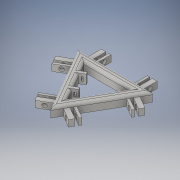
# Autodesk Inventor part: Test End effector
Saved by Autodesk Inventor 2016 (Build 200138000, 138)
## iProperties
Created: 2018-08-18
Part Number: Test End effector
Material: Generic
Document SubType Name: Modeling
Designer: Jorian Bruslind
Density: 1 g/cm^3
Appearance: Default
Author: Jorian Bruslind
Autodesk Inventor part; units mm, degrees
ref_plane "YZ Plane" through (0, 0, 0) normal (1, 0, 0) x (0, 1, 0)
ref_plane "XZ Plane" through (0, 0, 0) normal (0, 1, 0) x (-1, 0, 0)
ref_plane "XY Plane" through (0, 0, 0) normal (0, 0, 1) x (1, 0, 0)
sketch "Sketch1" plane through (0, 0, 0) normal (0, 1, 0) x (-1, 0, 0)
  line L0 (0, 46.188) -> (40, -23.094)
  line L1 (40, -23.094) -> (-40, -23.094)
  line L2 (-40, -23.094) -> (0, 46.188)
  line L3 (0, 28.8675) -> (25, -14.4338)
  line L4 (25, -14.4338) -> (-25, -14.4338)
  line L5 (-25, -14.4338) -> (0, 28.8675)
  point P0 (0, 0)
  point P1 (0, 0)
  point P2 (0, 0)
  dimension "d18" = 80
  dimension "d19" = 50
  constraints: 12 end point, 2 coincident, 14 other
  measures "d18" distance of L0.end L1.end
  measures "d19" distance of L3.end L4.end
extrude "Extrusion1" add sketch "Sketch1" along normal blind 10
sketch "Sketch5" plane through (40, 0, -23.094) normal (0.8660254, 0, 0.5) x (0.5, 0, -0.8660254)
  line L0 (0, 0) -> (-80, 0) projected
  line L1 (0, 0) -> (-10, 0)
  line L2 (-10, 0) -> (-15, 0)
  line L3 (-15, 0) -> (-15, 7)
  line L4 (-15, 7) -> (-10, 7)
  line L5 (-10, 7) -> (-10, 0)
  line L6 (-15, 0) -> (-18, 0)
  line L7 (-18, 0) -> (-20.5, 0)
  line L8 (-20.5, 0) -> (-20.5, 7)
  line L9 (-20.5, 7) -> (-18, 7)
  line L10 (-18, 7) -> (-18, 0)
  line L11 (-80, 0) -> (-70, 0)
  line L12 (-80, 0) -> (-40, 0) projected
  line L13 (-70, 0) -> (-65, 0)
  line L14 (-65, 0) -> (-65, 7)
  line L15 (-65, 7) -> (-70, 7)
  line L16 (-70, 7) -> (-70, 0)
  line L17 (-65, 0) -> (-62, 0)
  line L18 (-62, 0) -> (-59.5, 0)
  line L19 (-59.5, 0) -> (-59.5, 7)
  line L20 (-59.5, 7) -> (-62, 7)
  line L21 (-62, 7) -> (-62, 0)
  dimension "d44" = 10
  dimension "d45" = 5
  dimension "d46" = 7
  dimension "d47" = 3
  dimension "d48" = 2.5
  dimension "d49" = 10
  dimension "d50" = 5
  dimension "d51" = 7
  dimension "d52" = 3
  dimension "d53" = 2.5
  dimension "d54" = 7
  constraints: 40 end point, 8 parallel, 4 horizontal, 4 perpendicular, 4 point on line
  measures "d44" distance of L0.start L1.end
  measures "d45" distance of L3.end L4.end
  measures "d46" distance of L2.end L3.end
  measures "d47" distance of L2.end L6.end
  measures "d48" distance of L8.end L9.end
  measures "d49" distance of L0.end L11.end
  measures "d50" distance of L15.end L14.end
  measures "d51" distance of L14.end L13.end
  measures "d52" distance of L13.end L17.end
  measures "d53" distance of L20.end L19.end
  measures "d54" distance of L19.end L18.end
extrude "Extrusion3" add sketch "Sketch5" along normal blind 15
sketch "Sketch6" plane through (5, 0, 37.5278) normal (-0.5, 0, 0.8660254) x (0.8660254, 0, 0.5)
  line L0 (15, 0) -> (15, 7) projected
  line L1 (15, 3.5) -> (7.5, 3.5)
  circle A0 centre (7.5, 3.5) radius 2.25
  point P0 (-23.094, 0)
  dimension "d57" = 7.5
  dimension "d58" = 4.5
  constraints: 2 end point, 1 centre point, 1 coincident, 1 horizontal, 1 midpoint
  measures "d57" distance of L1.start L1.end
  measures "d58" diameter of A0
extrude "Extrusion4" cut sketch "Sketch6" against normal blind 60
sketch "Sketch7" plane through (0, 0, 46.188) normal (-0.8660254, 0, 0.5) x (0.5, 0, 0.8660254)
  line L0 (-80, 0) -> (-40, 0) projected
  line L1 (-80, 0) -> (-70, 0)
  line L2 (0, 0) -> (0, 10) projected
  line L3 (0, 0) -> (-10, 0)
  line L4 (0, 0) -> (-80, 0) projected
  line L5 (-70, 0) -> (-65, 0)
  line L6 (-65, 0) -> (-65, 7)
  line L7 (-65, 7) -> (-70, 7)
  line L8 (-70, 7) -> (-70, 0)
  line L9 (-65, 0) -> (-62, 0)
  line L10 (-65, 0) -> (-15, 0) projected
  line L11 (-62, 0) -> (-59.5, 0)
  line L12 (-59.5, 0) -> (-59.5, 7)
  line L13 (-59.5, 7) -> (-62, 7)
  line L14 (-62, 7) -> (-62, 0)
  line L15 (-10, 0) -> (-15, 0)
  line L16 (-15, 0) -> (-15, 7)
  line L17 (-15, 7) -> (-10, 7)
  line L18 (-10, 7) -> (-10, 0)
  line L19 (-15, 0) -> (-18, 0)
  line L20 (-32.5, 7) -> (-19.5096, 7) projected
  line L21 (-18, 0) -> (-20.5, 0)
  line L22 (-20.5, 0) -> (-20.5, 7)
  line L23 (-20.5, 7) -> (-18, 7)
  line L24 (-18, 7) -> (-18, 0)
  dimension "d61" = 10
  dimension "d62" = 10
  dimension "d63" = 5
  dimension "d64" = 7
  dimension "d65" = 3
  dimension "d66" = 2.5
  dimension "d67" = 7
  dimension "d68" = 5
  dimension "d69" = 7
  dimension "d70" = 3
  dimension "d71" = 2.5
  constraints: 40 end point, 8 parallel, 5 point on line, 4 horizontal, 4 perpendicular
  measures "d61" distance of L0.start L1.end
  measures "d62" distance of L2.start L3.end
  measures "d63" distance of L7.end L6.end
  measures "d64" distance of L6.end L5.end
  measures "d65" distance of L5.end L9.end
  measures "d66" distance of L13.end L12.end
  measures "d67" distance of L12.end L11.end
  measures "d68" distance of L16.end L17.end
  measures "d69" distance of L15.end L16.end
  measures "d70" distance of L15.end L19.end
  measures "d71" distance of L22.end L23.end
extrude "Extrusion5" add sketch "Sketch7" along normal blind 15
sketch "Sketch8" plane through (-35, 0, -14.4338) normal (-0.5, 0, -0.8660254) x (-0.8660254, 0, 0.5)
  line L0 (15, 7) -> (15, 0) projected
  line L1 (15, 3.5) -> (7.5, 3.5)
  circle A0 centre (7.5, 3.5) radius 2.25
  point P0 (-23.094, 0)
  dimension "d74" = 7.5
  dimension "d75" = 90
  dimension "d76" = 4.5
  constraints: 2 end point, 1 centre point, 1 coincident, 1 midpoint
  measures "d74" distance of L1.start L1.end
  measures "d75" angle of L0 L1
  measures "d76" diameter of A0
extrude "Extrusion6" cut sketch "Sketch8" against normal blind 60
sketch "Sketch9" plane through (40, 0, -23.094) normal (0, 0, -1) x (-1, 0, 0)
  line L0 (0, 0) -> (0, 10) projected
  line L1 (0, 0) -> (10, 0)
  line L2 (10.25, 0) -> (-2.7404, 0) projected
  line L3 (80, 0) -> (80, 10) projected
  line L4 (80, 0) -> (70, 0)
  line L5 (71, 0) -> (83.9904, 0) projected
  line L6 (10.25, 0) -> (15.25, 0)
  line L7 (15.25, 0) -> (15.25, 7)
  line L8 (15.25, 7) -> (10.25, 7)
  line L9 (10.25, 7) -> (10.25, 0)
  line L10 (15.25, 0) -> (18.25, 0)
  line L11 (18.0096, 0) -> (16.7596, 0) projected
  line L12 (32.5, 7) -> (19.5096, 7) projected
  line L13 (18.0096, 0) -> (20.5096, 0)
  line L14 (20.5096, 0) -> (20.5096, 7)
  line L15 (20.5096, 7) -> (18.0096, 7)
  line L16 (18.0096, 7) -> (18.0096, 0)
  line L17 (70, 0) -> (65, 0)
  line L18 (65, 0) -> (65, 7)
  line L19 (65, 7) -> (70, 7)
  line L20 (70, 7) -> (70, 0)
  line L21 (65, 0) -> (62, 0)
  line L22 (62, 0) -> (59.5, 0)
  line L23 (59.5, 0) -> (59.5, 7)
  line L24 (59.5, 7) -> (62, 7)
  line L25 (62, 7) -> (62, 0)
  point P0 (40, 0)
  dimension "d79" = 10
  dimension "d80" = 10
  dimension "d81" = 5
  dimension "d82" = 7
  dimension "d83" = 3
  dimension "d84" = 2.5
  dimension "d85" = 5
  dimension "d86" = 7
  dimension "d87" = 3
  dimension "d88" = 2.5
  dimension "d89" = 7
  constraints: 40 end point, 8 parallel, 5 horizontal, 4 perpendicular, 3 collinear, 1 point on line
  measures "d79" distance of L0.start L1.end
  measures "d80" distance of L3.start L4.end
  measures "d81" distance of L8.end L7.end
  measures "d82" distance of L7.end L6.end
  measures "d83" distance of L6.end L10.end
  measures "d84" distance of L15.end L14.end
  measures "d85" distance of L18.end L19.end
  measures "d86" distance of L17.end L18.end
  measures "d87" distance of L17.end L21.end
  measures "d88" distance of L23.end L24.end
  measures "d89" distance of L22.end L23.end
extrude "Extrusion7" add sketch "Sketch9" along normal blind 15
sketch "Sketch10" plane through (29.75, 0, -23.094) normal (1, 0, 0) x (0, 0, -1)
  line L0 (15, 7) -> (15, 0) projected
  line L1 (15, 3.5) -> (7.5, 3.5)
  circle A0 centre (7.5, 3.5) radius 2.25
  point P0 (-23.094, 0)
  dimension "d92" = 7.5
  dimension "d93" = 4.5
  constraints: 2 end point, 1 centre point, 1 coincident, 1 horizontal, 1 midpoint
  measures "d92" distance of L1.start L1.end
  measures "d93" diameter of A0
extrude "Extrusion8" cut sketch "Sketch10" against normal blind 60
sketch "Sketch11" plane through (-25, 0, -14.4338) normal (0.8660254, 0, -0.5) x (-0.5, 0, -0.8660254)
  line L0 (-25, 0) -> (-16, 0)
  line L1 (0, 0) -> (-50, 0) projected
  line L2 (-25, 0) -> (-16, 0) construction
  line L3 (-25, 0) -> (-34, 0)
  line L4 (-25, 0) -> (-16, 0) construction
  line L5 (-50, 10) -> (0, 10) projected
  line L6 (-16, 0) -> (-13, 0)
  line L7 (-13, 0) -> (-13, 10)
  line L8 (-13, 10) -> (-16, 10)
  line L9 (-16, 10) -> (-16, 0)
  line L10 (-34, 0) -> (-37, 0)
  line L11 (-37, 0) -> (-37, 10)
  line L12 (-37, 10) -> (-34, 10)
  line L13 (-34, 10) -> (-34, 0)
  dimension "d97" = 9
  dimension "d98" = 0
  dimension "d99" = 9
  dimension "d100" = 180
  dimension "d101" = 3
  dimension "d102" = 3
  constraints: 24 end point, 4 collinear, 4 horizontal, 4 parallel, 2 perpendicular, 2 point on line
  measures "d97" distance of L0.start L0.end
  measures "d98" distance between parallel lines of L2 L0
  measures "d99" distance of L0.start L3.end
  measures "d100" angle of L4 L3
  measures "d101" distance of L8.end L7.end
  measures "d102" distance of L11.end L12.end
extrude "Extrusion9" add sketch "Sketch11" along normal blind 6 contours L9 L5 L7 L1 | L1 L11 L5 L13
sketch "Sketch12" plane through (-6.5, 0, 17.6092) normal (0.5, 0, 0.8660254) x (0.8660254, 0, -0.5)
  line L0 (0, 10) -> (6, 10) projected
  line L1 (6, 10) -> (6, 7)
  line L2 (6, 0) -> (6, 10) projected
  line L3 (6, 7) -> (4, 7)
  line L4 (4, 7) -> (2, 7)
  line L5 (2, 7) -> (2, 3)
  line L6 (2, 3) -> (4, 3)
  line L7 (4, 3) -> (4, 7)
  point P0 (14.4338, 0)
  dimension "d105" = 3
  dimension "d106" = 2
  dimension "d107" = 2
  dimension "d108" = 4
  constraints: 12 end point, 2 horizontal, 2 parallel, 1 perpendicular, 1 point on line
  measures "d105" distance of L0.end L1.end
  measures "d106" distance of L1.end L3.end
  measures "d107" distance of L6.end L5.end
  measures "d108" distance of L5.end L4.end
extrude "Extrusion10" cut sketch "Sketch12" against normal blind 25
fillet "Fillet1" radius 3 8 edges at (20, 10, 11.547) (12.5, 10, 7.2169) (-20, 10, 11.547) (-12.5, 10, 7.2169) (-3.25, 10, 23.2383) (0, 10, -14.4338) (-21.75, 10, -8.8046) (0, 10, -23.094)
body "Solid1"
